Autodesk Fusion 360 part; units mm, degrees
note: some values were not read from the file. Chosen so that the rebuilt part matches the saved one: which face or edge a step refers to; which bodies a step acts on; where a thread starts. Set by a fixed rule: which sketch regions a step uses.
(part 2 of 2)
thread "Thread7" "ISO Metric profile 16.0 M16x2 6H" major diameter 16.2505 minor diameter 14.0225 pitch 2 angle 60 modelled right hand crest width 0.5471 on face at (52, 40.6981, -2.5233) crest through (57.8333, 40, -2.4888) on bodies 11 in component "mount"
thread "Thread3" "ISO Metric profile 16.0 M16x2 6g" major diameter 15.822 minor diameter 13.534 pitch 2 angle 60 modelled right hand crest width 0.2847 on face at (-4.6533, -38.431, 13.3333) crest through (-4.6041, -39.2276, 4.5) on bodies 13 in component "bolt"
fillet "Fillet3" radius 5 6 edges at (16.0036, -43.1172, 2.5) (6.2867, -52.168, 2.5) (-6.4099, -48.2783, 2.5) (-9.3897, -35.3379, 2.5) (0.3272, -26.2872, 2.5) (13.0238, -30.1768, 2.5) on bodies 13 in component "bolt"
component "Front" placed x (1, 0, 0) y (0, 1, 0) z (0, 0, 1) at (0, 0, 0)
component "right" placed x (1, 0, 0) y (0, 1, 0) z (0, 0, 1) at (0, 0, 0)
component "Front(Mirror)" placed x (1, 0, 0) y (0, -1, 0) z (0, 0, -1) at (0, 80, 0)
component "right(Mirror)" placed x (-1, 0, 0) y (0, 1, 0) z (0, 0, -1) at (160, 0, 0)
component "base" placed x (1, 0, 0) y (0, 1, 0) z (0, 0, 1) at (0, 0, 0)
component "divider" placed x (1, 0, 0) y (0, 1, 0) z (0, 0, 1) at (0, 0, 0)
component "electronics cover" placed x (1, 0, 0) y (0, 1, 0) z (0, 0, 1) at (0, 0, 0)
component "Food cover" placed x (1, 0, 0) y (0, 1, 0) z (0, 0, 1) at (0, 0, 0)
component "hopper" placed x (1, 0, 0) y (0, 1, 0) z (0, 0, 1) at (0, 0, 0)
component "hatch door" placed x (1, 0, 0) y (0, 1, 0) z (0, 0, 1) at (0, 0, 0)
component "mount" placed x (1, 0, 0) y (0, 1, 0) z (0, 0, 1) at (0, 0, 0)
component "divider2" placed x (1, 0, 0) y (0, 1, 0) z (0, 0, 1) at (0, 0, 0)
component "bolt" placed x (1, 0, 0) y (0, 1, 0) z (0, 0, 1) at (0, 0, 0)
equation "d1 = length"
equation "length = 160 mm"
equation "width = 80 mm"
equation "height = 100 mm"
equation "ntabs_3 = 3"
equation "ntabs_5 = 5"
equation "thickness = 3 mm"
equation "d8 = height"
equation "d9 = thickness"
equation "d10 = thickness"
equation "d11 = thickness"
equation "d12 = length / ntabs_5"
equation "d13 = d12"
equation "d14 = d12"
equation "d15 = d12"
equation "d16 = height / ntabs_3"
equation "d17 = d16"
equation "d18 = thickness"
equation "d20 = width"
equation "d21 = thickness"
equation "d22 = thickness"
equation "d23 = thickness"
equation "d24 = width / ntabs_3"
equation "d25 = d24"
equation "d26 = height / ntabs_3"
equation "d27 = d26"
equation "d28 = thickness"
equation "d33 = thickness"
equation "d34 = thickness"
equation "d35 = width / ntabs_3"
equation "d36 = d35"
equation "d37 = height / ntabs_3"
equation "d38 = d37"
equation "d39 = thickness"
equation "d45 = thickness"
equation "d46 = thickness"
equation "d47 = ( height + 2 * thickness ) / ntabs_3"
equation "d48 = d47"
equation "d49 = width / ntabs_3"
equation "d50 = d49"
equation "d51 = -thickness"
equation "d53 = -thickness"
equation "d58 = 12.25 mm + 5 mm"
equation "d74 = 24.775 mm + 5 mm"
equation "d85 = thickness"
equation "d87 = length * ( 1 / 3 )"
equation "d89 = thickness"
equation "d92 = -thickness"
equation "d94 = -thickness"
equation "d119 = thickness"
equation "d121 = thickness"
equation "d122 = thickness"
equation "d125 = ( 57 / ntabs_3 ) * 1 mm"
equation "d126 = d125"
equation "d127 = ( 94 / ntabs_3 ) * 1 mm"
equation "d128 = d127"
equation "d152 = ( 16 / 2 ) * 1 mm + 3.5 mm"
equation "d161 = ( 25 / 2 ) * 1 mm"
equation "d162 = 16 mm + 3.5 mm"
equation "d163 = ( width - 2 * thickness ) / 2"
